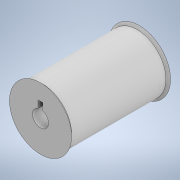
# Autodesk Inventor part: бабина
Saved by Autodesk Inventor 2021 (Build 250183000, 183)
## iProperties
Created: 2023-02-11
Part Number: бабина
Material: Типовые
Document SubType Name: Modeling
Designer: 1
Density: 1 g/cm^3
Appearance: По умолчанию
Author: 1
Autodesk Inventor part; units mm, degrees
ref_plane "YZ Plane" through (0, 0, 0) normal (1, 0, 0) x (0, 1, 0)
ref_plane "XZ Plane" through (0, 0, 0) normal (0, 1, 0) x (-1, 0, 0)
ref_plane "XY Plane" through (0, 0, 0) normal (0, 0, 1) x (1, 0, 0)
sketch "Эскиз1" plane through (0, 0, 0) normal (0, 0, 1) x (1, 0, 0)
  circle A0 centre (0, 0) radius 12.5
  circle A1 centre (0, 0) radius 3.5
  dimension "d0" = 25
  dimension "d1" = 7
  constraints: 2 centre point, 2 coincident
  measures "d0" diameter of A0
  measures "d1" diameter of A1
extrude "Выдавливание1" add sketch "Эскиз1" along normal mid plane 43
sketch "Эскиз2" plane through (0, 0, 21.5) normal (0, 0, 1) x (1, 0, 0)
  circle A0 centre (0, 0) radius 3.5 projected
  line L0 (-1, 3.3541) -> (1, 3.3541)
  line L1 (1, 3.3541) -> (1, 6.5)
  line L2 (1, 6.5) -> (-1, 6.5)
  line L3 (-1, 6.5) -> (-1, 3.3541)
  point P0 (0, 3.5)
  dimension "d4" = 3
  dimension "d5" = 2
  constraints: 8 end point, 3 point on circle, 2 parallel, 1 horizontal, 1 perpendicular, 1 vertical alignment
  measures "d4" distance from line of L2 point (0, 3.5)
  measures "d5" distance of L1.end L2.end
extrude "Выдавливание2" cut sketch "Эскиз2" against normal blind 22 contours L0 A0 | A0 L3 L2 L1 picked at (-0.1125, 3.3973)
sketch "Эскиз3" plane through (0, 0, 0) normal (1, 0, 0) x (0, 1, 0)
  line L0 (12.5, 21.5) -> (-12.5, 21.5) projected
  line L1 (12.5, 21.5) -> (13.5, 21.5)
  line L2 (13.5, 21.5) -> (12.5, 20.5)
  line L3 (12.5, 21.5) -> (12.5, 20.5)
  line L4 (12.5, -21.5) -> (12.5, 21.5) projected
  line L5 (0, 0) -> (17.3602, 0) construction
  line L6 (12.5, -21.5) -> (13.5, -21.5)
  line L7 (13.5, -21.5) -> (12.5, -20.5)
  line L8 (12.5, -21.5) -> (12.5, -20.5)
  line L9 (0, 0) -> (0, 32.2208)
  dimension "d8" = 1
  dimension "d9" = 45
  constraints: 16 end point, 4 symmetric about line, 2 horizontal, 1 point on line, 1 vertical
  measures "d8" distance of L0.start L1.end
  measures "d9" angle of L1 L2
revolve "Вращение1" add sketch "Эскиз3" angle 360 about axis through (0, 0, 0) along (0, 0, 1)
